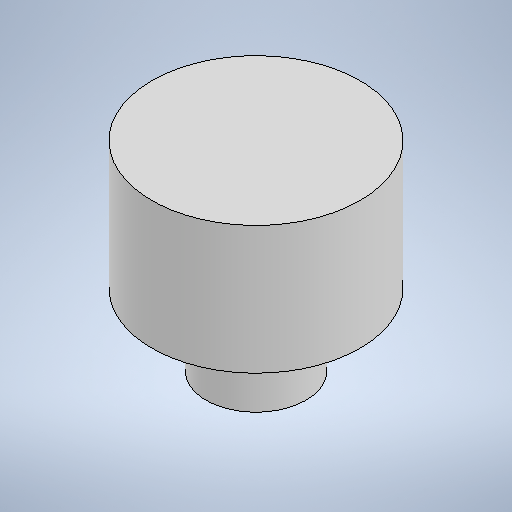
# Autodesk Inventor part: TKS dummy filter element
Saved by Autodesk Inventor 2025 (Build 290162010, 162A)
## iProperties
Created: 2025-07-02
Part Number: TKS dummy filter element
Material: Generic
Document SubType Name: Modeling
Designer: user
Density: 1 g/cm^3
Appearance: Default
Author: user
Autodesk Inventor part; units mm, degrees
ref_plane "YZ Plane" through (0, 0, 0) normal (1, 0, 0) x (0, 1, 0)
ref_plane "XZ Plane" through (0, 0, 0) normal (0, 1, 0) x (-1, 0, 0)
ref_plane "XY Plane" through (0, 0, 0) normal (0, 0, 1) x (1, 0, 0)
sketch "Sketch1" plane through (0, 0, 0) normal (0, 1, 0) x (-1, 0, 0)
  line L0 (0, 0) -> (0, 50)
  line L1 (0, 50) -> (-26, 50)
  line L2 (-26, 50) -> (-26, 18)
  line L3 (-26, 18) -> (-12.5, 15.6196)
  line L4 (-12.5, 15.6196) -> (-12.5, 0)
  line L5 (-12.5, 0) -> (0, 0)
  dimension "d0" = 50
  dimension "d1" = 52
  dimension "d2" = 25
  dimension "d3" = 32
  dimension "d4" = 100
  constraints: 12 end point, 2 perpendicular, 1 horizontal, 1 parallel, 1 vertical
  measures "d0" distance of L0.start L0.end
  measures "d1" diameter of L2 L0
  measures "d2" diameter of L4 L0
  measures "d3" distance from line of L2.end L1
  measures "d4" angle of L4 L3
revolve "Revolution1" add sketch "Sketch1" angle 360 about axis through (0, 0, 0) along (0, 0, 1)
body "Solid1"
